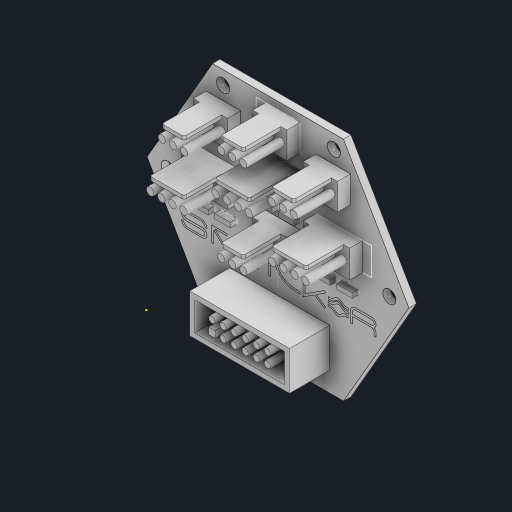
# Autodesk Inventor part: ArmControlBoardPcb
Saved by Autodesk Inventor 2023 (Build 270158000, 158)
## iProperties
Created: 2023-12-09
Part Number: ArmControlBoardPcb
Material: Generic
Document SubType Name: Modeling
Designer: valer
Density: 1 g/cm^3
Appearance: Default
Author: valer
Autodesk Inventor part; units mm, degrees
(part 1 of 3)
ref_plane "YZ Plane" through (0, 0, 0) normal (1, 0, 0) x (0, 1, 0)
ref_plane "XZ Plane" through (0, 0, 0) normal (0, 1, 0) x (-1, 0, 0)
ref_plane "XY Plane" through (0, 0, 0) normal (0, 0, 1) x (1, 0, 0)
sketch "Sketch1" plane through (0, 0, 0) normal (0, 0, 1) x (1, 0, 0)
  circle A0 centre (55.6982, 30.5264) radius 1.5
  line L0 (31.7743, 35.9084) -> (31.7952, 36.0136)
  line L1 (31.7952, 36.0136) -> (31.8548, 36.1028)
  line L2 (31.8548, 36.1028) -> (31.944, 36.1624)
  line L3 (31.944, 36.1624) -> (32.0493, 36.1834)
  line L4 (32.0493, 36.1834) -> (32.7493, 36.1834)
  line L5 (32.7493, 36.1834) -> (32.8545, 36.1624)
  line L6 (32.8545, 36.1624) -> (32.9437, 36.1028)
  line L7 (32.9437, 36.1028) -> (33.0033, 36.0136)
  line L8 (33.0033, 36.0136) -> (33.0243, 35.9084)
  line L9 (33.0243, 35.9084) -> (33.0243, 35.3584)
  line L10 (33.0243, 35.3584) -> (33.0033, 35.2531)
  line L11 (33.0033, 35.2531) -> (32.9437, 35.1639)
  line L12 (32.9437, 35.1639) -> (32.8545, 35.1043)
  line L13 (32.8545, 35.1043) -> (32.7493, 35.0834)
  line L14 (32.7493, 35.0834) -> (32.0493, 35.0834)
  line L15 (32.0493, 35.0834) -> (31.944, 35.1043)
  line L16 (31.944, 35.1043) -> (31.8548, 35.1639)
  line L17 (31.8548, 35.1639) -> (31.7952, 35.2531)
  line L18 (31.7952, 35.2531) -> (31.7743, 35.3584)
  line L19 (31.7743, 35.3584) -> (31.7743, 35.9084)
  line L20 (34.1243, 35.9084) -> (34.1452, 36.0136)
  line L21 (34.1452, 36.0136) -> (34.2048, 36.1028)
  line L22 (34.2048, 36.1028) -> (34.294, 36.1624)
  line L23 (34.294, 36.1624) -> (34.3993, 36.1834)
  line L24 (34.3993, 36.1834) -> (35.0993, 36.1834)
  line L25 (35.0993, 36.1834) -> (35.2045, 36.1624)
  line L26 (35.2045, 36.1624) -> (35.2937, 36.1028)
  line L27 (35.2937, 36.1028) -> (35.3533, 36.0136)
  line L28 (35.3533, 36.0136) -> (35.3743, 35.9084)
  line L29 (35.3743, 35.9084) -> (35.3743, 35.3584)
  line L30 (35.3743, 35.3584) -> (35.3533, 35.2531)
  line L31 (35.3533, 35.2531) -> (35.2937, 35.1639)
  line L32 (35.2937, 35.1639) -> (35.2045, 35.1043)
  line L33 (35.2045, 35.1043) -> (35.0993, 35.0834)
  line L34 (35.0993, 35.0834) -> (34.3993, 35.0834)
  line L35 (34.3993, 35.0834) -> (34.294, 35.1043)
  line L36 (34.294, 35.1043) -> (34.2048, 35.1639)
  line L37 (34.2048, 35.1639) -> (34.1452, 35.2531)
  line L38 (34.1452, 35.2531) -> (34.1243, 35.3584)
  line L39 (34.1243, 35.3584) -> (34.1243, 35.9084)
  line L40 (40.0232, 28.2614) -> (40.0441, 28.3666)
  line L41 (40.0441, 28.3666) -> (40.1037, 28.4558)
  line L42 (40.1037, 28.4558) -> (40.1929, 28.5154)
  line L43 (40.1929, 28.5154) -> (40.2982, 28.5364)
  line L44 (40.2982, 28.5364) -> (40.9982, 28.5364)
  line L45 (40.9982, 28.5364) -> (41.1034, 28.5154)
  line L46 (41.1034, 28.5154) -> (41.1926, 28.4558)
  line L47 (41.1926, 28.4558) -> (41.2522, 28.3666)
  line L48 (41.2522, 28.3666) -> (41.2732, 28.2614)
  line L49 (41.2732, 28.2614) -> (41.2732, 27.7114)
  line L50 (41.2732, 27.7114) -> (41.2522, 27.6061)
  line L51 (41.2522, 27.6061) -> (41.1926, 27.5169)
  line L52 (41.1926, 27.5169) -> (41.1034, 27.4573)
  line L53 (41.1034, 27.4573) -> (40.9982, 27.4364)
  line L54 (40.9982, 27.4364) -> (40.2982, 27.4364)
  line L55 (40.2982, 27.4364) -> (40.1929, 27.4573)
  line L56 (40.1929, 27.4573) -> (40.1037, 27.5169)
  line L57 (40.1037, 27.5169) -> (40.0441, 27.6061)
  line L58 (40.0441, 27.6061) -> (40.0232, 27.7114)
  line L59 (40.0232, 27.7114) -> (40.0232, 28.2614)
  line L60 (42.3732, 28.2614) -> (42.3941, 28.3666)
  line L61 (42.3941, 28.3666) -> (42.4537, 28.4558)
  line L62 (42.4537, 28.4558) -> (42.5429, 28.5154)
  line L63 (42.5429, 28.5154) -> (42.6482, 28.5364)
  line L64 (42.6482, 28.5364) -> (43.3482, 28.5364)
  line L65 (43.3482, 28.5364) -> (43.4534, 28.5154)
  line L66 (43.4534, 28.5154) -> (43.5426, 28.4558)
  line L67 (43.5426, 28.4558) -> (43.6022, 28.3666)
  line L68 (43.6022, 28.3666) -> (43.6232, 28.2614)
  line L69 (43.6232, 28.2614) -> (43.6232, 27.7114)
  line L70 (43.6232, 27.7114) -> (43.6022, 27.6061)
  line L71 (43.6022, 27.6061) -> (43.5426, 27.5169)
  line L72 (43.5426, 27.5169) -> (43.4534, 27.4573)
  line L73 (43.4534, 27.4573) -> (43.3482, 27.4364)
  line L74 (43.3482, 27.4364) -> (42.6482, 27.4364)
  line L75 (42.6482, 27.4364) -> (42.5429, 27.4573)
  line L76 (42.5429, 27.4573) -> (42.4537, 27.5169)
  line L77 (42.4537, 27.5169) -> (42.3941, 27.6061)
  line L78 (42.3941, 27.6061) -> (42.3732, 27.7114)
  line L79 (42.3732, 27.7114) -> (42.3732, 28.2614)
  circle A1 centre (40.4582, 35.6064) radius 0.8763
  circle A2 centre (42.9982, 35.6064) radius 0.8763
  circle A3 centre (45.5382, 35.6064) radius 0.8763
  circle A4 centre (48.0782, 35.6064) radius 0.8763
  line L80 (45.1032, 28.2614) -> (45.1241, 28.3666)
  line L81 (45.1241, 28.3666) -> (45.1837, 28.4558)
  line L82 (45.1837, 28.4558) -> (45.2729, 28.5154)
  line L83 (45.2729, 28.5154) -> (45.3782, 28.5364)
  line L84 (45.3782, 28.5364) -> (46.0782, 28.5364)
  line L85 (46.0782, 28.5364) -> (46.1834, 28.5154)
  line L86 (46.1834, 28.5154) -> (46.2726, 28.4558)
  line L87 (46.2726, 28.4558) -> (46.3322, 28.3666)
  line L88 (46.3322, 28.3666) -> (46.3532, 28.2614)
  line L89 (46.3532, 28.2614) -> (46.3532, 27.7114)
  line L90 (46.3532, 27.7114) -> (46.3322, 27.6061)
  line L91 (46.3322, 27.6061) -> (46.2726, 27.5169)
  line L92 (46.2726, 27.5169) -> (46.1834, 27.4573)
  line L93 (46.1834, 27.4573) -> (46.0782, 27.4364)
  line L94 (46.0782, 27.4364) -> (45.3782, 27.4364)
  line L95 (45.3782, 27.4364) -> (45.2729, 27.4573)
  line L96 (45.2729, 27.4573) -> (45.1837, 27.5169)
  line L97 (45.1837, 27.5169) -> (45.1241, 27.6061)
  line L98 (45.1241, 27.6061) -> (45.1032, 27.7114)
  line L99 (45.1032, 27.7114) -> (45.1032, 28.2614)
  line L100 (47.4532, 28.2614) -> (47.4741, 28.3666)
  line L101 (47.4741, 28.3666) -> (47.5337, 28.4558)
  line L102 (47.5337, 28.4558) -> (47.6229, 28.5154)
  line L103 (47.6229, 28.5154) -> (47.7282, 28.5364)
  line L104 (47.7282, 28.5364) -> (48.4282, 28.5364)
  line L105 (48.4282, 28.5364) -> (48.5334, 28.5154)
  line L106 (48.5334, 28.5154) -> (48.6226, 28.4558)
  line L107 (48.6226, 28.4558) -> (48.6822, 28.3666)
  line L108 (48.6822, 28.3666) -> (48.7032, 28.2614)
  line L109 (48.7032, 28.2614) -> (48.7032, 27.7114)
  line L110 (48.7032, 27.7114) -> (48.6822, 27.6061)
  line L111 (48.6822, 27.6061) -> (48.6226, 27.5169)
  line L112 (48.6226, 27.5169) -> (48.5334, 27.4573)
  line L113 (48.5334, 27.4573) -> (48.4282, 27.4364)
  line L114 (48.4282, 27.4364) -> (47.7282, 27.4364)
  line L115 (47.7282, 27.4364) -> (47.6229, 27.4573)
  line L116 (47.6229, 27.4573) -> (47.5337, 27.5169)
  line L117 (47.5337, 27.5169) -> (47.4741, 27.6061)
  line L118 (47.4741, 27.6061) -> (47.4532, 27.7114)
  line L119 (47.4532, 27.7114) -> (47.4532, 28.2614)
  line L120 (28.5429, 6.4763) -> (28.5638, 6.5815)
  line L121 (28.5638, 6.5815) -> (28.6234, 6.6707)
  line L122 (28.6234, 6.6707) -> (28.7126, 6.7303)
  line L123 (28.7126, 6.7303) -> (28.8179, 6.7513)
  line L124 (28.8179, 6.7513) -> (29.5179, 6.7513)
  line L125 (29.5179, 6.7513) -> (29.6231, 6.7303)
  line L126 (29.6231, 6.7303) -> (29.7123, 6.6707)
  line L127 (29.7123, 6.6707) -> (29.7719, 6.5815)
  line L128 (29.7719, 6.5815) -> (29.7929, 6.4763)
  line L129 (29.7929, 6.4763) -> (29.7929, 5.9263)
  line L130 (29.7929, 5.9263) -> (29.7719, 5.821)
  line L131 (29.7719, 5.821) -> (29.7123, 5.7318)
  line L132 (29.7123, 5.7318) -> (29.6231, 5.6722)
  line L133 (29.6231, 5.6722) -> (29.5179, 5.6513)
  line L134 (29.5179, 5.6513) -> (28.8179, 5.6513)
  line L135 (28.8179, 5.6513) -> (28.7126, 5.6722)
  line L136 (28.7126, 5.6722) -> (28.6234, 5.7318)
  line L137 (28.6234, 5.7318) -> (28.5638, 5.821)
  line L138 (28.5638, 5.821) -> (28.5429, 5.9263)
  line L139 (28.5429, 5.9263) -> (28.5429, 6.4763)
  line L140 (30.8929, 6.4763) -> (30.9138, 6.5815)
  line L141 (30.9138, 6.5815) -> (30.9734, 6.6707)
  line L142 (30.9734, 6.6707) -> (31.0626, 6.7303)
  line L143 (31.0626, 6.7303) -> (31.1679, 6.7513)
  line L144 (31.1679, 6.7513) -> (31.8679, 6.7513)
  line L145 (31.8679, 6.7513) -> (31.9731, 6.7303)
  line L146 (31.9731, 6.7303) -> (32.0623, 6.6707)
  line L147 (32.0623, 6.6707) -> (32.1219, 6.5815)
  line L148 (32.1219, 6.5815) -> (32.1429, 6.4763)
  line L149 (32.1429, 6.4763) -> (32.1429, 5.9263)
  line L150 (32.1429, 5.9263) -> (32.1219, 5.821)
  line L151 (32.1219, 5.821) -> (32.0623, 5.7318)
  line L152 (32.0623, 5.7318) -> (31.9731, 5.6722)
  line L153 (31.9731, 5.6722) -> (31.8679, 5.6513)
  line L154 (31.8679, 5.6513) -> (31.1679, 5.6513)
  line L155 (31.1679, 5.6513) -> (31.0626, 5.6722)
  line L156 (31.0626, 5.6722) -> (30.9734, 5.7318)
  line L157 (30.9734, 5.7318) -> (30.9138, 5.821)
  line L158 (30.9138, 5.821) -> (30.8929, 5.9263)
  line L159 (30.8929, 5.9263) -> (30.8929, 6.4763)
  circle A5 centre (27.4699, 42.6062) radius 0.8763
  circle A6 centre (30.0099, 42.6062) radius 0.8763
  circle A7 centre (32.5499, 42.6062) radius 0.8763
  circle A8 centre (35.0899, 42.6062) radius 0.8763
  circle A9 centre (40.3371, 47.4317) radius 0.8509
  circle A10 centre (42.8771, 47.4317) radius 0.8509
  circle A11 centre (45.4171, 47.4317) radius 0.8509
  line L160 (23.5019, 11.5158) -> (23.5019, 13.0058)
  line L161 (23.5019, 13.0058) -> (24.9919, 13.0058)
  line L162 (24.9919, 13.0058) -> (24.9919, 11.5158)
  line L163 (24.9919, 11.5158) -> (23.5019, 11.5158)
  circle A12 centre (24.2469, 14.8008) radius 0.745
  circle A13 centre (26.7869, 12.2608) radius 0.745
  circle A14 centre (26.7869, 14.8008) radius 0.745
  circle A15 centre (29.3269, 12.2608) radius 0.745
  circle A16 centre (29.3269, 14.8008) radius 0.745
  circle A17 centre (31.8669, 12.2608) radius 0.745
  circle A18 centre (31.8669, 14.8008) radius 0.745
  circle A19 centre (34.4069, 12.2608) radius 0.745
  circle A20 centre (34.4069, 14.8008) radius 0.745
  circle A21 centre (36.9469, 12.2608) radius 0.745
  circle A22 centre (36.9469, 14.8008) radius 0.745
  line L164 (12.0832, 28.2614) -> (12.1041, 28.3666) construction
  line L165 (12.1041, 28.3666) -> (12.1637, 28.4558) construction
  line L166 (12.1637, 28.4558) -> (12.2529, 28.5154) construction
  line L167 (12.2529, 28.5154) -> (12.3582, 28.5364) construction
  line L168 (12.3582, 28.5364) -> (13.0582, 28.5364) construction
  line L169 (13.0582, 28.5364) -> (13.1634, 28.5154) construction
  line L170 (13.1634, 28.5154) -> (13.2526, 28.4558) construction
  line L171 (13.2526, 28.4558) -> (13.3122, 28.3666) construction
  line L172 (13.3122, 28.3666) -> (13.3332, 28.2614) construction
  line L173 (13.3332, 28.2614) -> (13.3332, 27.7114) construction
  line L174 (13.3332, 27.7114) -> (13.3122, 27.6061) construction
  line L175 (13.3122, 27.6061) -> (13.2526, 27.5169) construction
  line L176 (13.2526, 27.5169) -> (13.1634, 27.4573) construction
  line L177 (13.1634, 27.4573) -> (13.0582, 27.4364) construction
  line L178 (13.0582, 27.4364) -> (12.3582, 27.4364) construction
  line L179 (12.3582, 27.4364) -> (12.2529, 27.4573) construction
  line L180 (12.2529, 27.4573) -> (12.1637, 27.5169) construction
  line L181 (12.1637, 27.5169) -> (12.1041, 27.6061) construction
  line L182 (12.1041, 27.6061) -> (12.0832, 27.7114) construction
  line L183 (12.0832, 27.7114) -> (12.0832, 28.2614) construction
  line L184 (14.4332, 28.2614) -> (14.4541, 28.3666) construction
  line L185 (14.4541, 28.3666) -> (14.5137, 28.4558) construction
  line L186 (14.5137, 28.4558) -> (14.6029, 28.5154) construction
  line L187 (14.6029, 28.5154) -> (14.7082, 28.5364) construction
  line L188 (14.7082, 28.5364) -> (15.4082, 28.5364) construction
  line L189 (15.4082, 28.5364) -> (15.5134, 28.5154) construction
  line L190 (15.5134, 28.5154) -> (15.6026, 28.4558) construction
  line L191 (15.6026, 28.4558) -> (15.6622, 28.3666) construction
  line L192 (15.6622, 28.3666) -> (15.6832, 28.2614) construction
  line L193 (15.6832, 28.2614) -> (15.6832, 27.7114) construction
  line L194 (15.6832, 27.7114) -> (15.6622, 27.6061) construction
  line L195 (15.6622, 27.6061) -> (15.6026, 27.5169) construction
  line L196 (15.6026, 27.5169) -> (15.5134, 27.4573) construction
  line L197 (15.5134, 27.4573) -> (15.4082, 27.4364) construction
  line L198 (15.4082, 27.4364) -> (14.7082, 27.4364) construction
  line L199 (14.7082, 27.4364) -> (14.6029, 27.4573) construction
  line L200 (14.6029, 27.4573) -> (14.5137, 27.5169) construction
  line L201 (14.5137, 27.5169) -> (14.4541, 27.6061) construction
  line L202 (14.4541, 27.6061) -> (14.4332, 27.7114) construction
  line L203 (14.4332, 27.7114) -> (14.4332, 28.2614) construction
  circle A23 centre (28.7399, 51.8275) radius 0.8509
  circle A24 centre (31.2799, 51.8275) radius 0.8509
  circle A25 centre (33.8199, 51.8275) radius 0.8509
  line L204 (17.1632, 28.2614) -> (17.1841, 28.3666) construction
  line L205 (17.1841, 28.3666) -> (17.2437, 28.4558) construction
  line L206 (17.2437, 28.4558) -> (17.3329, 28.5154) construction
  line L207 (17.3329, 28.5154) -> (17.4382, 28.5364) construction
  line L208 (17.4382, 28.5364) -> (18.1382, 28.5364)
  line L209 (18.1382, 28.5364) -> (18.2434, 28.5154) construction
  line L210 (18.2434, 28.5154) -> (18.3326, 28.4558) construction
  line L211 (18.3326, 28.4558) -> (18.3922, 28.3666) construction
  line L212 (18.3922, 28.3666) -> (18.4132, 28.2614) construction
  line L213 (18.4132, 28.2614) -> (18.4132, 27.7114) construction
  line L214 (18.4132, 27.7114) -> (18.3922, 27.6061) construction
  line L215 (18.3922, 27.6061) -> (18.3326, 27.5169) construction
  line L216 (18.3326, 27.5169) -> (18.2434, 27.4573) construction
  line L217 (18.2434, 27.4573) -> (18.1382, 27.4364) construction
  line L218 (18.1382, 27.4364) -> (17.4382, 27.4364) construction
  line L219 (17.4382, 27.4364) -> (17.3329, 27.4573) construction
  line L220 (17.3329, 27.4573) -> (17.2437, 27.5169) construction
  line L221 (17.2437, 27.5169) -> (17.1841, 27.6061) construction
  line L222 (17.1841, 27.6061) -> (17.1632, 27.7114) construction
  line L223 (17.1632, 27.7114) -> (17.1632, 28.2614) construction
  line L224 (19.5132, 28.2614) -> (19.5341, 28.3666) construction
  line L225 (19.5341, 28.3666) -> (19.5937, 28.4558) construction
  line L226 (19.5937, 28.4558) -> (19.6829, 28.5154) construction
  line L227 (19.6829, 28.5154) -> (19.7882, 28.5364) construction
  line L228 (19.7882, 28.5364) -> (20.4882, 28.5364) construction
  line L229 (20.4882, 28.5364) -> (20.5934, 28.5154) construction
  line L230 (20.5934, 28.5154) -> (20.6826, 28.4558) construction
  line L231 (20.6826, 28.4558) -> (20.7422, 28.3666) construction
  line L232 (20.7422, 28.3666) -> (20.7632, 28.2614) construction
  line L233 (20.7632, 28.2614) -> (20.7632, 27.7114) construction
  line L234 (20.7632, 27.7114) -> (20.7422, 27.6061) construction
  line L235 (20.7422, 27.6061) -> (20.6826, 27.5169) construction
  line L236 (20.6826, 27.5169) -> (20.5934, 27.4573) construction
  line L237 (20.5934, 27.4573) -> (20.4882, 27.4364) construction
  line L238 (20.4882, 27.4364) -> (19.7882, 27.4364) construction
  line L239 (19.7882, 27.4364) -> (19.6829, 27.4573) construction
  line L240 (19.6829, 27.4573) -> (19.5937, 27.5169) construction
  line L241 (19.5937, 27.5169) -> (19.5341, 27.6061) construction
  line L242 (19.5341, 27.6061) -> (19.5132, 27.7114) construction
  line L243 (19.5132, 27.7114) -> (19.5132, 28.2614) construction
  circle A26 centre (28.7399, 30.5264) radius 0.8509
  circle A27 centre (31.2799, 30.5264) radius 0.8509
  circle A28 centre (33.8199, 30.5264) radius 0.8509
  line L244 (29.4649, 26.3259) -> (29.4858, 26.4311)
  line L245 (29.4858, 26.4311) -> (29.5454, 26.5203)
  line L246 (29.5454, 26.5203) -> (29.6346, 26.5799)
  line L247 (29.6346, 26.5799) -> (29.7399, 26.6009)
  line L248 (29.7399, 26.6009) -> (30.4399, 26.6009)
  line L249 (30.4399, 26.6009) -> (30.5451, 26.5799)
  line L250 (30.5451, 26.5799) -> (30.6343, 26.5203)
  line L251 (30.6343, 26.5203) -> (30.6939, 26.4311)
  line L252 (30.6939, 26.4311) -> (30.7149, 26.3259)
  line L253 (30.7149, 26.3259) -> (30.7149, 25.7759)
  line L254 (30.7149, 25.7759) -> (30.6939, 25.6706)
  line L255 (30.6939, 25.6706) -> (30.6343, 25.5814)
  line L256 (30.6343, 25.5814) -> (30.5451, 25.5218)
  line L257 (30.5451, 25.5218) -> (30.4399, 25.5009)
  line L258 (30.4399, 25.5009) -> (29.7399, 25.5009)
  line L259 (29.7399, 25.5009) -> (29.6346, 25.5218)
  line L260 (29.6346, 25.5218) -> (29.5454, 25.5814)
  line L261 (29.5454, 25.5814) -> (29.4858, 25.6706)
  line L262 (29.4858, 25.6706) -> (29.4649, 25.7759)
  line L263 (29.4649, 25.7759) -> (29.4649, 26.3259)
  line L264 (31.8149, 26.3259) -> (31.8358, 26.4311)
  line L265 (31.8358, 26.4311) -> (31.8954, 26.5203)
  line L266 (31.8954, 26.5203) -> (31.9846, 26.5799)
  line L267 (31.9846, 26.5799) -> (32.0899, 26.6009)
  line L268 (32.0899, 26.6009) -> (32.7899, 26.6009)
  line L269 (32.7899, 26.6009) -> (32.8951, 26.5799)
  line L270 (32.8951, 26.5799) -> (32.9843, 26.5203)
  line L271 (32.9843, 26.5203) -> (33.0439, 26.4311)
  line L272 (33.0439, 26.4311) -> (33.0649, 26.3259)
  line L273 (33.0649, 25.7759) -> (33.0439, 25.6706)
  line L274 (33.0439, 25.6706) -> (32.9843, 25.5814)
  line L275 (32.9843, 25.5814) -> (32.8951, 25.5218)
  line L276 (32.8951, 25.5218) -> (32.7899, 25.5009)
  line L277 (32.7899, 25.5009) -> (32.0899, 25.5009)
  line L278 (32.0899, 25.5009) -> (31.9846, 25.5218)
  line L279 (31.9846, 25.5218) -> (31.8954, 25.5814)
  line L280 (31.8954, 25.5814) -> (31.8358, 25.6706)
  line L281 (31.8358, 25.6706) -> (31.8149, 25.7759)
  line L282 (31.8149, 25.7759) -> (31.8149, 26.3259)
  circle A29 centre (12.5182, 35.6064) radius 0.8763
  circle A30 centre (15.0582, 35.6064) radius 0.8763
  circle A31 centre (17.5982, 35.6064) radius 0.8763
  circle A32 centre (20.1382, 35.6064) radius 0.8763
  line L283 (26.6943, 35.9084) -> (26.7152, 36.0136)
  line L284 (26.7152, 36.0136) -> (26.7748, 36.1028)
  line L285 (26.7748, 36.1028) -> (26.864, 36.1624)
  line L286 (26.864, 36.1624) -> (26.9693, 36.1834)
  line L287 (26.9693, 36.1834) -> (27.6693, 36.1834)
  line L288 (27.6693, 36.1834) -> (27.7745, 36.1624)
  line L289 (27.7745, 36.1624) -> (27.8637, 36.1028)
  line L290 (27.8637, 36.1028) -> (27.9233, 36.0136)
  line L291 (27.9233, 36.0136) -> (27.9443, 35.9084)
  line L292 (27.9443, 35.9084) -> (27.9443, 35.3584)
  line L293 (27.9443, 35.3584) -> (27.9233, 35.2531)
  line L294 (27.9233, 35.2531) -> (27.8637, 35.1639)
  line L295 (27.8637, 35.1639) -> (27.7745, 35.1043)
  line L296 (27.7745, 35.1043) -> (27.6693, 35.0834)
  line L297 (27.6693, 35.0834) -> (26.9693, 35.0834)
  line L298 (26.9693, 35.0834) -> (26.864, 35.1043)
  line L299 (26.864, 35.1043) -> (26.7748, 35.1639)
  line L300 (26.7748, 35.1639) -> (26.7152, 35.2531)
  line L301 (26.7152, 35.2531) -> (26.6943, 35.3584)
  line L302 (26.6943, 35.3584) -> (26.6943, 35.9084)
  line L303 (29.0443, 35.9084) -> (29.0652, 36.0136)
  line L304 (29.0652, 36.0136) -> (29.1248, 36.1028)
  line L305 (29.1248, 36.1028) -> (29.214, 36.1624)
  line L306 (29.214, 36.1624) -> (29.3193, 36.1834)
  line L307 (29.3193, 36.1834) -> (30.0193, 36.1834)
  line L308 (30.0193, 36.1834) -> (30.1245, 36.1624)
  line L309 (30.1245, 36.1624) -> (30.2137, 36.1028)
  line L310 (30.2137, 36.1028) -> (30.2733, 36.0136)
  line L311 (30.2733, 36.0136) -> (30.2943, 35.9084)
  line L312 (30.2943, 35.9084) -> (30.2943, 35.3584)
  line L313 (30.2943, 35.3584) -> (30.2733, 35.2531)
  line L314 (30.2733, 35.2531) -> (30.2137, 35.1639)
  line L315 (30.2137, 35.1639) -> (30.1245, 35.1043)
  line L316 (30.1245, 35.1043) -> (30.0193, 35.0834)
  line L317 (30.0193, 35.0834) -> (29.3193, 35.0834)
  line L318 (29.3193, 35.0834) -> (29.214, 35.1043)
  line L319 (29.214, 35.1043) -> (29.1248, 35.1639)
  line L320 (29.1248, 35.1639) -> (29.0652, 35.2531)
  line L321 (29.0652, 35.2531) -> (29.0443, 35.3584)
  line L322 (29.0443, 35.3584) -> (29.0443, 35.9084)
  circle A33 centre (15.1689, 47.3537) radius 0.8509
  circle A34 centre (17.7089, 47.3537) radius 0.8509
  circle A35 centre (20.2489, 47.3537) radius 0.8509
  line L323 (20.1652, 35.6334) -> (20.1382, 35.6064)
  line L324 (26.4028, 18.3787) -> (26.4027, 18.3787)
  line L325 (44.019, 24.3143) -> (44.055, 24.3125)
  line L326 (44.055, 24.3125) -> (44.0904, 24.3095)
  line L327 (44.0904, 24.3095) -> (44.125, 24.3055)
  line L328 (44.125, 24.3055) -> (44.159, 24.3003)
  line L329 (44.159, 24.3003) -> (44.1923, 24.2942)
  line L330 (44.1923, 24.2942) -> (44.257, 24.2789)
  line L331 (44.257, 24.2789) -> (44.3195, 24.2602)
  line L332 (44.3195, 24.2602) -> (44.3798, 24.2382)
  line L333 (44.3798, 24.2382) -> (44.4381, 24.2133)
  line L334 (44.4381, 24.2133) -> (44.4948, 24.1859)
  line L335 (44.4948, 24.1859) -> (44.5498, 24.1564)
  line L336 (44.5498, 24.1564) -> (44.6035, 24.125)
  line L337 (44.6035, 24.125) -> (44.6561, 24.0922)
  line L338 (44.6561, 24.0922) -> (44.7077, 24.0582)
  line L339 (44.7077, 24.0582) -> (44.8087, 23.9883)
  line L340 (44.8087, 23.9883) -> (44.9082, 23.918)
  line L341 (44.9082, 23.918) -> (45.1198, 23.7816)
  line L342 (45.1198, 23.7816) -> (45.2244, 23.718)
  line L343 (45.2244, 23.718) -> (45.2775, 23.6882)
  line L344 (45.2775, 23.6882) -> (45.3315, 23.6601)
  line L345 (45.3315, 23.6601) -> (45.3867, 23.6337)
  line L346 (45.3867, 23.6337) -> (45.4435, 23.6095)
  line L347 (45.4435, 23.6095) -> (45.5022, 23.5876)
  line L348 (45.5022, 23.5876) -> (45.563, 23.5683)
  line L349 (45.563, 23.5683) -> (45.6263, 23.5517)
  line L350 (45.6263, 23.5517) -> (45.6924, 23.5382)
  line L351 (45.6924, 23.5382) -> (45.7616, 23.5279)
  line L352 (45.7616, 23.5279) -> (45.8342, 23.5212)
  line L353 (45.8342, 23.5212) -> (46.3369, 23.5212)
  line L354 (46.3369, 23.5212) -> (46.3369, 23.0714)
  line L355 (46.3369, 23.0714) -> (45.8342, 23.0714)
  line L356 (45.8342, 23.0714) -> (45.7851, 23.0722)
  line L357 (45.7851, 23.0722) -> (45.7371, 23.0747)
  line L358 (45.7371, 23.0747) -> (45.6902, 23.0787)
  line L359 (45.6902, 23.0787) -> (45.6442, 23.0843)
  line L360 (45.6442, 23.0843) -> (45.5992, 23.0913)
  line L361 (45.5992, 23.0913) -> (45.5552, 23.0996)
  line L362 (45.5552, 23.0996) -> (45.5121, 23.1093)
  line L363 (45.5121, 23.1093) -> (45.47, 23.1202)
  line L364 (45.47, 23.1202) -> (45.4287, 23.1322)
  line L365 (45.4287, 23.1322) -> (45.3883, 23.1453)
  line L366 (45.3883, 23.1453) -> (45.3101, 23.1746)
  line L367 (45.3101, 23.1746) -> (45.2349, 23.2075)
  line L368 (45.2349, 23.2075) -> (45.1628, 23.2433)
  line L369 (45.1628, 23.2433) -> (45.0935, 23.2817)
  line L370 (45.0935, 23.2817) -> (45.0268, 23.322)
  line L371 (45.0268, 23.322) -> (44.9624, 23.3637)
  line L372 (44.9624, 23.3637) -> (44.9003, 23.4062)
  line L373 (44.9003, 23.4062) -> (44.7819, 23.4917)
  line L374 (44.7819, 23.4917) -> (44.67, 23.5741)
  line L375 (44.67, 23.5741) -> (44.583, 23.6409)
  line L376 (44.583, 23.6409) -> (44.4997, 23.7018)
  line L377 (44.4997, 23.7018) -> (44.4591, 23.7298)
  line L378 (44.4591, 23.7298) -> (44.4189, 23.7559)
  line L379 (44.4189, 23.7559) -> (44.379, 23.7801)
  line L380 (44.379, 23.7801) -> (44.3393, 23.8023)
  line L381 (44.3393, 23.8023) -> (44.2996, 23.8223)
  line L382 (44.2996, 23.8223) -> (44.2597, 23.84)
  line L383 (44.2597, 23.84) -> (44.2195, 23.8552)
  line L384 (44.2195, 23.8552) -> (44.1789, 23.868)
  line L385 (44.1789, 23.868) -> (44.1376, 23.8781)
  line L386 (44.1376, 23.8781) -> (44.0956, 23.8855)
  line L387 (44.0956, 23.8855) -> (44.0526, 23.89)
  line L388 (44.0526, 23.89) -> (44.0086, 23.8916)
  line L389 (44.0086, 23.8916) -> (43.9645, 23.89)
  line L390 (43.9645, 23.89) -> (43.9216, 23.8855)
  line L391 (43.9216, 23.8855) -> (43.8795, 23.8781)
  line L392 (43.8795, 23.8781) -> (43.8383, 23.868)
  line L393 (43.8383, 23.868) -> (43.7976, 23.8552)
  line L394 (43.7976, 23.8552) -> (43.7574, 23.84)
  line L395 (43.7574, 23.84) -> (43.7176, 23.8223)
  line L396 (43.7176, 23.8223) -> (43.6779, 23.8023)
  line L397 (43.6779, 23.8023) -> (43.6381, 23.7801)
  line L398 (43.6381, 23.7801) -> (43.5983, 23.7559)
  line L399 (43.5983, 23.7559) -> (43.5581, 23.7298)
  line L400 (43.5581, 23.7298) -> (43.5174, 23.7018)
  line L401 (43.5174, 23.7018) -> (43.4341, 23.6409)
  line L402 (43.4341, 23.6409) -> (43.3471, 23.5741)
  line L403 (43.3471, 23.5741) -> (43.2352, 23.4841)
  line L404 (43.2352, 23.4841) -> (43.1169, 23.3951)
  line L405 (43.1169, 23.3951) -> (43.0547, 23.352)
  line L406 (43.0547, 23.352) -> (42.9904, 23.3104)
  line L407 (42.9904, 23.3104) -> (42.9237, 23.2707)
  line L408 (42.9237, 23.2707) -> (42.8543, 23.2334)
  line L409 (42.8543, 23.2334) -> (42.7822, 23.1989)
  line L410 (42.7822, 23.1989) -> (42.7071, 23.1676)
  line L411 (42.7071, 23.1676) -> (42.6288, 23.14)
  line L412 (42.6288, 23.14) -> (42.5472, 23.1164)
  line L413 (42.5472, 23.1164) -> (42.462, 23.0974)
  line L414 (42.462, 23.0974) -> (42.373, 23.0832)
  line L415 (42.373, 23.0832) -> (42.28, 23.0744)
  line L416 (42.28, 23.0744) -> (42.183, 23.0714)
  line L417 (42.183, 23.0714) -> (41.6803, 23.0714)
  line L418 (41.6803, 23.0714) -> (41.6803, 23.5212)
  line L419 (41.6803, 23.5212) -> (42.183, 23.5212)
  line L420 (42.183, 23.5212) -> (42.215, 23.5218)
  line L421 (42.215, 23.5218) -> (42.2465, 23.5236)
  line L422 (42.2465, 23.5236) -> (42.2777, 23.5265)
  line L423 (42.2777, 23.5265) -> (42.3084, 23.5306)
  line L424 (42.3084, 23.5306) -> (42.3387, 23.5358)
  line L425 (42.3387, 23.5358) -> (42.3686, 23.5419)
  line L426 (42.3686, 23.5419) -> (42.4273, 23.5571)
  line L427 (42.4273, 23.5571) -> (42.4846, 23.5759)
  line L428 (42.4846, 23.5759) -> (42.5406, 23.5979)
  line L429 (42.5406, 23.5979) -> (42.5955, 23.6228)
  line L430 (42.5955, 23.6228) -> (42.6493, 23.6501)
  line L431 (42.6493, 23.6501) -> (42.7022, 23.6797)
  line L432 (42.7022, 23.6797) -> (42.7542, 23.7111)
  line L433 (42.7542, 23.7111) -> (42.8056, 23.7439)
  line L434 (42.8056, 23.7439) -> (42.8564, 23.7779)
  line L435 (42.8564, 23.7779) -> (43.0561, 23.918)
  line L436 (43.0561, 23.918) -> (43.1556, 23.9959)
  line L437 (43.1556, 23.9959) -> (43.2058, 24.0333)
  line L438 (43.2058, 24.0333) -> (43.2566, 24.0693)
  line L439 (43.2566, 24.0693) -> (43.3082, 24.1039)
  line L440 (43.3082, 24.1039) -> (43.3607, 24.1366)
  line L441 (43.3607, 24.1366) -> (43.4144, 24.1674)
  line L442 (43.4144, 24.1674) -> (43.4695, 24.1958)
  line L443 (43.4695, 24.1958) -> (43.5261, 24.2219)
  line L444 (43.5261, 24.2219) -> (43.5845, 24.2451)
  line L445 (43.5845, 24.2451) -> (43.6448, 24.2655)
  line L446 (43.6448, 24.2655) -> (43.7072, 24.2827)
  line L447 (43.7072, 24.2827) -> (43.772, 24.2964)
  line L448 (43.772, 24.2964) -> (43.8392, 24.3065)
  line L449 (43.8392, 24.3065) -> (43.9092, 24.3128)
  line L450 (43.9092, 24.3128) -> (43.9821, 24.3149)
  line L451 (43.9821, 24.3149) -> (44.019, 24.3143)
  line L452 (18.5028, 23.971) -> (15.7246, 23.971)
  line L453 (15.7246, 23.971) -> (18.635, 21.087)
  line L454 (18.635, 21.087) -> (18.344, 20.7695)
  line L455 (18.344, 20.7695) -> (15.4336, 23.6535)
  line L456 (15.4336, 23.6535) -> (15.4336, 20.8753)
  line L457 (15.4336, 20.8753) -> (14.9838, 20.8753)
  line L458 (14.9838, 20.8753) -> (14.9838, 24.3943)
  line L459 (14.9838, 24.3943) -> (18.5028, 24.3943)
  line L460 (18.5028, 24.3943) -> (18.5028, 23.971)
  line L461 (51.3988, 24.4192) -> (51.4835, 24.4146)
  line L462 (51.4835, 24.4146) -> (51.5652, 24.407)
  line L463 (51.5652, 24.407) -> (51.6439, 24.3964)
  line L464 (51.6439, 24.3964) -> (51.7196, 24.3828)
  line L465 (51.7196, 24.3828) -> (51.7925, 24.3663)
  line L466 (51.7925, 24.3663) -> (51.8624, 24.347)
  line L467 (51.8624, 24.347) -> (51.9295, 24.3248)
  line L468 (51.9295, 24.3248) -> (51.9939, 24.2999)
  line L469 (51.9939, 24.2999) -> (52.0555, 24.2722)
  line L470 (52.0555, 24.2722) -> (52.1144, 24.2418)
  line L471 (52.1144, 24.2418) -> (52.1706, 24.2087)
  line L472 (52.1706, 24.2087) -> (52.2241, 24.1729)
  line L473 (52.2241, 24.1729) -> (52.2751, 24.1346)
  line L474 (52.2751, 24.1346) -> (52.3235, 24.0937)
  line L475 (52.3235, 24.0937) -> (52.3694, 24.0503)
  line L476 (52.3694, 24.0503) -> (52.3935, 24.0254)
  line L477 (52.3935, 24.0254) -> (52.416, 24.0002)
  line L478 (52.416, 24.0002) -> (52.4371, 23.9748)
  line L479 (52.4371, 23.9748) -> (52.4567, 23.9493)
  line L480 (52.4567, 23.9493) -> (52.4751, 23.9237)
  line L481 (52.4751, 23.9237) -> (52.4921, 23.8982)
  line L482 (52.4921, 23.8982) -> (52.5078, 23.8727)
  line L483 (52.5078, 23.8727) -> (52.5224, 23.8473)
  line L484 (52.5224, 23.8473) -> (52.5358, 23.8222)
  line L485 (52.5358, 23.8222) -> (52.548, 23.7973)
  line L486 (52.548, 23.7973) -> (52.5592, 23.7727)
  line L487 (52.5592, 23.7727) -> (52.5694, 23.7485)
  line L488 (52.5694, 23.7485) -> (52.5869, 23.7015)
  line L489 (52.5869, 23.7015) -> (52.6009, 23.6568)
  line L490 (52.6009, 23.6568) -> (52.6118, 23.6148)
  line L491 (52.6118, 23.6148) -> (52.62, 23.5762)
  line L492 (52.62, 23.5762) -> (52.6259, 23.5414)
  line L493 (52.6259, 23.5414) -> (52.6299, 23.5108)
  line L494 (52.6299, 23.5108) -> (52.6323, 23.4851)
  line L495 (52.6323, 23.4851) -> (52.6335, 23.4647)
  line L496 (52.6335, 23.4647) -> (52.634, 23.4418)
  line L497 (52.634, 23.4418) -> (52.634, 23.336)
  line L498 (52.634, 23.336) -> (52.6299, 23.2785)
  line L499 (52.6299, 23.2785) -> (52.6259, 23.2489)
  line L500 (52.6259, 23.2489) -> (52.62, 23.2146)
  line L501 (52.62, 23.2146) -> (52.6118, 23.1761)
  line L502 (52.6118, 23.1761) -> (52.6009, 23.1342)
  line L503 (52.6009, 23.1342) -> (52.5869, 23.0895)
  line L504 (52.5869, 23.0895) -> (52.5694, 23.0427)
  line L505 (52.5694, 23.0427) -> (52.548, 22.9944)
  line L506 (52.548, 22.9944) -> (52.5224, 22.9453)
  line L507 (52.5224, 22.9453) -> (52.4921, 22.896)
  line L508 (52.4921, 22.896) -> (52.4751, 22.8715)
  line L509 (52.4751, 22.8715) -> (52.4567, 22.8472)
  line L510 (52.4567, 22.8472) -> (52.4371, 22.8233)
  line L511 (52.4371, 22.8233) -> (52.416, 22.7996)
  line L512 (52.416, 22.7996) -> (52.3935, 22.7765)
  line L513 (52.3935, 22.7765) -> (52.3694, 22.7539)
  line L514 (52.3694, 22.7539) -> (52.3293, 22.7142)
  line L515 (52.3293, 22.7142) -> (52.3085, 22.6943)
  line L516 (52.3085, 22.6943) -> (52.2867, 22.6745)
  line L517 (52.2867, 22.6745) -> (52.2637, 22.6546)
  line L518 (52.2637, 22.6546) -> (52.2517, 22.6447)
  line L519 (52.2517, 22.6447) -> (52.2392, 22.6348)
  line L520 (52.2392, 22.6348) -> (52.2262, 22.6249)
  line L521 (52.2262, 22.6249) -> (52.2128, 22.615)
  line L522 (52.2128, 22.615) -> (52.1988, 22.605)
  line L523 (52.1988, 22.605) -> (52.1842, 22.5951)
  line L524 (52.1842, 22.5951) -> (52.1988, 22.5852)
  line L525 (52.1988, 22.5852) -> (52.2128, 22.5753)
  line L526 (52.2128, 22.5753) -> (52.2262, 22.5654)
  line L527 (52.2262, 22.5654) -> (52.2392, 22.5554)
  line L528 (52.2392, 22.5554) -> (52.2517, 22.5455)
  line L529 (52.2517, 22.5455) -> (52.2637, 22.5356)
  line L530 (52.2637, 22.5356) -> (52.2754, 22.5257)
  line L531 (52.2754, 22.5257) -> (52.2867, 22.5157)
  line L532 (52.2867, 22.5157) -> (52.3085, 22.4959)
  line L533 (52.3085, 22.4959) -> (52.3293, 22.4761)
  line L534 (52.3293, 22.4761) -> (52.3495, 22.4562)
  line L535 (52.3495, 22.4562) -> (52.3694, 22.4364)
  line L536 (52.3694, 22.4364) -> (52.3935, 22.4114)
  line L537 (52.3935, 22.4114) -> (52.416, 22.3862)
  line L538 (52.416, 22.3862) -> (52.4371, 22.3608)
  line L539 (52.4371, 22.3608) -> (52.4567, 22.3353)
  line L540 (52.4567, 22.3353) -> (52.4751, 22.3098)
  line L541 (52.4751, 22.3098) -> (52.4921, 22.2842)
  line L542 (52.4921, 22.2842) -> (52.5078, 22.2587)
  line L543 (52.5078, 22.2587) -> (52.5224, 22.2334)
  line L544 (52.5224, 22.2334) -> (52.5358, 22.2082)
  line L545 (52.5358, 22.2082) -> (52.548, 22.1833)
  line L546 (52.548, 22.1833) -> (52.5592, 22.1587)
  line L547 (52.5592, 22.1587) -> (52.5694, 22.1345)
  line L548 (52.5694, 22.1345) -> (52.5869, 22.0875)
  line L549 (52.5869, 22.0875) -> (52.6009, 22.0428)
  line L550 (52.6009, 22.0428) -> (52.6118, 22.0009)
  line L551 (52.6118, 22.0009) -> (52.62, 21.9622)
  line L552 (52.62, 21.9622) -> (52.6259, 21.9274)
  line L553 (52.6259, 21.9274) -> (52.6299, 21.8969)
  line L554 (52.6299, 21.8969) -> (52.6323, 21.8711)
  line L555 (52.6323, 21.8711) -> (52.6335, 21.8507)
  line L556 (52.6335, 21.8507) -> (52.634, 21.8278)
  line L557 (52.634, 21.8278) -> (52.634, 20.8753)
  line L558 (52.634, 20.8753) -> (52.1842, 20.8753)
  line L559 (52.1842, 20.8753) -> (52.1842, 21.8278)
  line L560 (52.1842, 21.8278) -> (52.1825, 21.8658)
  line L561 (52.1825, 21.8658) -> (52.1785, 21.8963)
  line L562 (52.1785, 21.8963) -> (52.1706, 21.9328)
  line L563 (52.1706, 21.9328) -> (52.1576, 21.974)
  line L564 (52.1576, 21.974) -> (52.1382, 22.0185)
  line L565 (52.1382, 22.0185) -> (52.1111, 22.065)
  line L566 (52.1111, 22.065) -> (52.0943, 22.0886)
  line L567 (52.0943, 22.0886) -> (52.0751, 22.1123)
  line L568 (52.0751, 22.1123) -> (52.0533, 22.1357)
  line L569 (52.0533, 22.1357) -> (52.0288, 22.1589)
  line L570 (52.0288, 22.1589) -> (52.0014, 22.1815)
  line L571 (52.0014, 22.1815) -> (51.971, 22.2035)
  line L572 (51.971, 22.2035) -> (51.9374, 22.2247)
  line L573 (51.9374, 22.2247) -> (51.9005, 22.2449)
  line L574 (51.9005, 22.2449) -> (51.86, 22.264)
  line L575 (51.86, 22.264) -> (51.8159, 22.2818)
  line L576 (51.8159, 22.2818) -> (51.7679, 22.298)
  line L577 (51.7679, 22.298) -> (51.7159, 22.3127)
  line L578 (51.7159, 22.3127) -> (51.6597, 22.3255)
  line L579 (51.6597, 22.3255) -> (51.5993, 22.3364)
  line L580 (51.5993, 22.3364) -> (51.5343, 22.3452)
  line L581 (51.5343, 22.3452) -> (51.4648, 22.3516)
  line L582 (51.4648, 22.3516) -> (51.3904, 22.3556)
  line L583 (51.3904, 22.3556) -> (51.3111, 22.357)
  line L584 (51.3111, 22.357) -> (47.263, 22.357)
  line L585 (47.263, 22.357) -> (47.263, 20.8753)
  line L586 (47.263, 20.8753) -> (46.8132, 20.8753)
  line L587 (46.8132, 20.8753) -> (46.8132, 22.8068)
  line L588 (47.263, 22.8068) -> (51.3111, 22.8068)
  line L589 (51.3111, 22.8068) -> (51.3743, 22.8074)
  line L590 (51.3743, 22.8074) -> (51.4352, 22.8094)
  line L591 (51.4352, 22.8094) -> (51.4936, 22.8127)
  line L592 (51.4936, 22.8127) -> (51.5496, 22.8175)
  line L593 (51.5496, 22.8175) -> (51.6033, 22.8239)
  line L594 (51.6033, 22.8239) -> (51.6548, 22.8319)
  line L595 (51.6548, 22.8319) -> (51.704, 22.8416)
  line L596 (51.704, 22.8416) -> (51.751, 22.8531)
  line L597 (51.751, 22.8531) -> (51.7958, 22.8664)
  line L598 (51.7958, 22.8664) -> (51.8384, 22.8817)
  line L599 (51.8384, 22.8817) -> (51.879, 22.899)
  line L600 (51.879, 22.899) -> (51.9176, 22.9184)
  line L601 (51.9176, 22.9184) -> (51.9541, 22.94)
  line L602 (51.9541, 22.94) -> (51.9886, 22.9638)
  line L603 (51.9886, 22.9638) -> (52.0212, 22.9899)
  line L604 (52.0212, 22.9899) -> (52.0519, 23.0185)
  line L605 (52.0519, 23.0185) -> (52.0663, 23.0286)
  line L606 (52.0663, 23.0286) -> (52.0799, 23.0392)
  line L607 (52.0799, 23.0392) -> (52.0925, 23.0501)
  line L608 (52.0925, 23.0501) -> (52.1043, 23.0613)
  line L609 (52.1043, 23.0613) -> (52.1153, 23.0729)
  line L610 (52.1153, 23.0729) -> (52.1255, 23.0846)
  line L611 (52.1255, 23.0846) -> (52.135, 23.0965)
  line L612 (52.135, 23.0965) -> (52.1437, 23.1086)
  line L613 (52.1437, 23.1086) -> (52.1517, 23.1207)
  line L614 (52.1517, 23.1207) -> (52.1591, 23.1328)
  line L615 (52.1591, 23.1328) -> (52.1658, 23.145)
  line L616 (52.1658, 23.145) -> (52.1719, 23.157)
  line L617 (52.1719, 23.157) -> (52.1774, 23.169)
  line L618 (52.1774, 23.169) -> (52.1824, 23.1808)
  line L619 (52.1824, 23.1808) -> (52.1869, 23.1924)
  line L620 (52.1869, 23.1924) -> (52.1908, 23.2037)
  line L621 (52.1908, 23.2037) -> (52.1974, 23.2253)
  line L622 (52.1974, 23.2253) -> (52.2023, 23.2453)
  line L623 (52.2023, 23.2453) -> (52.2058, 23.2633)
  line L624 (52.2058, 23.2633) -> (52.2082, 23.2789)
  line L625 (52.2082, 23.2789) -> (52.2096, 23.2917)
  line L626 (52.2096, 23.2917) -> (52.2104, 23.3013)
  line L627 (52.2104, 23.3013) -> (52.2107, 23.3095)
  line L628 (52.2107, 23.3095) -> (52.2107, 23.4153)
  line L629 (52.2107, 23.4153) -> (52.209, 23.4533)
  line L630 (52.209, 23.4533) -> (52.2049, 23.4838)
  line L631 (52.2049, 23.4838) -> (52.197, 23.5203)
  line L632 (52.197, 23.5203) -> (52.184, 23.5615)
  line L633 (52.184, 23.5615) -> (52.1646, 23.606)
  line L634 (52.1646, 23.606) -> (52.1376, 23.6525)
  line L635 (52.1376, 23.6525) -> (52.1207, 23.6761)
  line L636 (52.1207, 23.6761) -> (52.1015, 23.6998)
  line L637 (52.1015, 23.6998) -> (52.0798, 23.7232)
  line L638 (52.0798, 23.7232) -> (52.0553, 23.7464)
  line L639 (52.0553, 23.7464) -> (52.0279, 23.769)
  line L640 (52.0279, 23.769) -> (51.9975, 23.791)
  line L641 (51.9975, 23.791) -> (51.9639, 23.8122)
  line L642 (51.9639, 23.8122) -> (51.9269, 23.8324)
  line L643 (51.9269, 23.8324) -> (51.8865, 23.8515)
  line L644 (51.8865, 23.8515) -> (51.8423, 23.8693)
  line L645 (51.8423, 23.8693) -> (51.7943, 23.8855)
  line L646 (51.7943, 23.8855) -> (51.7423, 23.9002)
  line L647 (51.7423, 23.9002) -> (51.6862, 23.913)
  line L648 (51.6862, 23.913) -> (51.6257, 23.9239)
  line L649 (51.6257, 23.9239) -> (51.5608, 23.9327)
  line L650 (51.5608, 23.9327) -> (51.4912, 23.9391)
  line L651 (51.4912, 23.9391) -> (51.4169, 23.9431)
  line L652 (51.4169, 23.9431) -> (51.3375, 23.9445)
  line L653 (51.3375, 23.9445) -> (48.1625, 23.9445)
  line L654 (48.1625, 23.9445) -> (48.0993, 23.9439)
  line L655 (48.0993, 23.9439) -> (48.0385, 23.9419)
  line L656 (48.0385, 23.9419) -> (47.9801, 23.9386)
  line L657 (47.9801, 23.9386) -> (47.924, 23.9337)
  line L658 (47.924, 23.9337) -> (47.8703, 23.9274)
  line L659 (47.8703, 23.9274) -> (47.8188, 23.9194)
  line L660 (47.8188, 23.9194) -> (47.7697, 23.9097)
  line L661 (47.7697, 23.9097) -> (47.7227, 23.8982)
  line L662 (47.7227, 23.8982) -> (47.6779, 23.8848)
  line L663 (47.6779, 23.8848) -> (47.6352, 23.8696)
  line L664 (47.6352, 23.8696) -> (47.5946, 23.8523)
  line L665 (47.5946, 23.8523) -> (47.5561, 23.8329)
  line L666 (47.5561, 23.8329) -> (47.5196, 23.8113)
  line L667 (47.5196, 23.8113) -> (47.485, 23.7875)
  line L668 (47.485, 23.7875) -> (47.4524, 23.7614)
  line L669 (47.4524, 23.7614) -> (47.4217, 23.7328)
  line L670 (47.4217, 23.7328) -> (47.4073, 23.7227)
  line L671 (47.4073, 23.7227) -> (47.3938, 23.7121)
  line L672 (47.3938, 23.7121) -> (47.3811, 23.7012)
  line L673 (47.3811, 23.7012) -> (47.3693, 23.6899)
  line L674 (47.3693, 23.6899) -> (47.3583, 23.6784)
  line L675 (47.3583, 23.6784) -> (47.3481, 23.6667)
  line L676 (47.3481, 23.6667) -> (47.3387, 23.6547)
  line L677 (47.3387, 23.6547) -> (47.3299, 23.6427)
  line L678 (47.3299, 23.6427) -> (47.3219, 23.6306)
  line L679 (47.3219, 23.6306) -> (47.3145, 23.6184)
  line L680 (47.3145, 23.6184) -> (47.3078, 23.6063)
  line L681 (47.3078, 23.6063) -> (47.3017, 23.5942)
  line L682 (47.3017, 23.5942) -> (47.2962, 23.5823)
  line L683 (47.2962, 23.5823) -> (47.2912, 23.5705)
  line L684 (47.2912, 23.5705) -> (47.2868, 23.5589)
  line L685 (47.2868, 23.5589) -> (47.2828, 23.5476)
  line L686 (47.2828, 23.5476) -> (47.2763, 23.526)
  line L687 (47.2763, 23.526) -> (47.2713, 23.506)
  line L688 (47.2713, 23.506) -> (47.2678, 23.488)
  line L689 (47.2678, 23.488) -> (47.2654, 23.4724)
  line L690 (47.2654, 23.4724) -> (47.264, 23.4596)
  line L691 (47.264, 23.4596) -> (47.2633, 23.4499)
  line L692 (47.2633, 23.4499) -> (47.263, 23.4418)
  line L693 (47.263, 23.4418) -> (47.263, 22.8068)
  line L694 (46.8132, 22.8068) -> (46.8132, 23.4418)
  line L695 (46.8132, 23.4418) -> (46.8173, 23.4997)
  line L696 (46.8173, 23.4997) -> (46.8271, 23.5646)
  line L697 (46.8271, 23.5646) -> (46.8353, 23.6038)
  line L698 (46.8353, 23.6038) -> (46.8462, 23.6468)
  line L699 (46.8462, 23.6468) -> (46.8603, 23.6929)
  line L700 (46.8603, 23.6929) -> (46.8778, 23.7415)
  line L701 (46.8778, 23.7415) -> (46.8991, 23.7919)
  line L702 (46.8991, 23.7919) -> (46.9248, 23.8436)
  line L703 (46.9248, 23.8436) -> (46.9551, 23.8959)
  line L704 (46.9551, 23.8959) -> (46.9904, 23.9482)
  line L705 (46.9904, 23.9482) -> (47.0101, 23.9742)
  line L706 (47.0101, 23.9742) -> (47.0312, 23.9999)
  line L707 (47.0312, 23.9999) -> (47.0537, 24.0253)
  line L708 (47.0537, 24.0253) -> (47.0778, 24.0503)
  line L709 (47.0778, 24.0503) -> (47.1236, 24.0937)
  line L710 (47.1236, 24.0937) -> (47.1721, 24.1346)
  line L711 (47.1721, 24.1346) -> (47.223, 24.1729)
  line L712 (47.223, 24.1729) -> (47.2766, 24.2087)
  line L713 (47.2766, 24.2087) -> (47.3328, 24.2418)
  line L714 (47.3328, 24.2418) -> (47.3917, 24.2722)
  line L715 (47.3917, 24.2722) -> (47.4533, 24.2999)
  line L716 (47.4533, 24.2999) -> (47.5176, 24.3248)
  line L717 (47.5176, 24.3248) -> (47.5848, 24.347)
  line L718 (47.5848, 24.347) -> (47.6547, 24.3663)
  line L719 (47.6547, 24.3663) -> (47.7275, 24.3828)
  line L720 (47.7275, 24.3828) -> (47.8033, 24.3964)
  line L721 (47.8033, 24.3964) -> (47.882, 24.407)
  line L722 (47.882, 24.407) -> (47.9636, 24.4146)
  line L723 (47.9636, 24.4146) -> (48.0483, 24.4192)
  line L724 (48.0483, 24.4192) -> (48.1361, 24.4207)
  line L725 (48.1361, 24.4207) -> (51.3111, 24.4207)
  line L726 (51.3111, 24.4207) -> (51.3988, 24.4192)
  line L727 (24.3587, 24.4192) -> (24.4442, 24.4146)
  line L728 (24.4442, 24.4146) -> (24.527, 24.407)
  line L729 (24.527, 24.407) -> (24.6072, 24.3964)
  line L730 (24.6072, 24.3964) -> (24.6845, 24.3828)
  line L731 (24.6845, 24.3828) -> (24.759, 24.3663)
  line L732 (24.759, 24.3663) -> (24.8305, 24.347)
  line L733 (24.8305, 24.347) -> (24.8991, 24.3248)
  line L734 (24.8991, 24.3248) -> (24.9645, 24.2999)
  line L735 (24.9645, 24.2999) -> (25.0267, 24.2722)
  line L736 (25.0267, 24.2722) -> (25.0857, 24.2418)
  line L737 (25.0857, 24.2418) -> (25.1413, 24.2087)
  line L738 (25.1413, 24.2087) -> (25.1935, 24.1729)
  line L739 (25.1935, 24.1729) -> (25.2423, 24.1346)
  line L740 (25.2423, 24.1346) -> (25.2875, 24.0937)
  line L741 (25.2875, 24.0937) -> (25.329, 24.0503)
  line L742 (25.329, 24.0503) -> (25.353, 24.0254)
  line L743 (25.353, 24.0254) -> (25.3756, 24.0002)
  line L744 (25.3756, 24.0002) -> (25.3967, 23.9748)
  line L745 (25.3967, 23.9748) -> (25.4163, 23.9493)
  line L746 (25.4163, 23.9493) -> (25.4347, 23.9237)
  line L747 (25.4347, 23.9237) -> (25.4517, 23.8982)
  line L748 (25.4517, 23.8982) -> (25.4674, 23.8727)
  line L749 (25.4674, 23.8727) -> (25.482, 23.8473)
  line L750 (25.482, 23.8473) -> (25.4953, 23.8222)
  line L751 (25.4953, 23.8222) -> (25.5076, 23.7973)
  line L752 (25.5076, 23.7973) -> (25.5188, 23.7727)
  line L753 (25.5188, 23.7727) -> (25.529, 23.7485)
  line L754 (25.529, 23.7485) -> (25.5465, 23.7015)
  line L755 (25.5465, 23.7015) -> (25.5605, 23.6568)
  line L756 (25.5605, 23.6568) -> (25.5714, 23.6148)
  line L757 (25.5714, 23.6148) -> (25.5796, 23.5762)
  line L758 (25.5796, 23.5762) -> (25.5855, 23.5414)
  line L759 (25.5855, 23.5414) -> (25.5895, 23.5108)
  line L760 (25.5895, 23.5108) -> (25.5918, 23.4851)
  line L761 (25.5918, 23.4851) -> (25.5931, 23.4647)
  line L762 (25.5931, 23.4647) -> (25.5936, 23.4418)
  line L763 (25.5936, 23.4418) -> (25.5936, 23.336)
  line L764 (25.5936, 23.336) -> (25.5931, 23.3131)
  line L765 (25.5931, 23.3131) -> (25.5895, 23.2673)
  line L766 (25.5895, 23.2673) -> (25.5855, 23.2372)
  line L767 (25.5855, 23.2372) -> (25.5796, 23.2029)
  line L768 (25.5796, 23.2029) -> (25.5714, 23.1651)
  line L769 (25.5714, 23.1651) -> (25.5605, 23.1243)
  line L770 (25.5605, 23.1243) -> (25.5465, 23.081)
  line L771 (25.5465, 23.081) -> (25.529, 23.0357)
  line L772 (25.529, 23.0357) -> (25.5076, 22.9891)
  line L773 (25.5076, 22.9891) -> (25.482, 22.9416)
  line L774 (25.482, 22.9416) -> (25.4517, 22.8937)
  line L775 (25.4517, 22.8937) -> (25.4347, 22.8699)
  line L776 (25.4347, 22.8699) -> (25.4163, 22.8462)
  line L777 (25.4163, 22.8462) -> (25.3967, 22.8226)
  line L778 (25.3967, 22.8226) -> (25.3756, 22.7994)
  line L779 (25.3756, 22.7994) -> (25.353, 22.7764)
  line L780 (25.353, 22.7764) -> (25.329, 22.7539)
  line L781 (25.329, 22.7539) -> (25.2889, 22.7142)
  line L782 (25.2889, 22.7142) -> (25.2681, 22.6943)
  line L783 (25.2681, 22.6943) -> (25.2463, 22.6745)
  line L784 (25.2463, 22.6745) -> (25.2233, 22.6546)
  line L785 (25.2233, 22.6546) -> (25.2113, 22.6447)
  line L786 (25.2113, 22.6447) -> (25.1988, 22.6348)
  line L787 (25.1988, 22.6348) -> (25.1858, 22.6249)
  line L788 (25.1858, 22.6249) -> (25.1724, 22.615)
  line L789 (25.1724, 22.615) -> (25.1584, 22.605)
  line L790 (25.1584, 22.605) -> (25.1438, 22.5951)
  line L791 (25.1438, 22.5951) -> (25.1584, 22.5852)
  line L792 (25.1584, 22.5852) -> (25.1724, 22.5753)
  line L793 (25.1724, 22.5753) -> (25.1858, 22.5654)
  line L794 (25.1858, 22.5654) -> (25.1988, 22.5554)
  line L795 (25.1988, 22.5554) -> (25.2113, 22.5455)
  line L796 (25.2113, 22.5455) -> (25.2233, 22.5356)
  line L797 (25.2233, 22.5356) -> (25.235, 22.5257)
  line L798 (25.235, 22.5257) -> (25.2463, 22.5157)
  line L799 (25.2463, 22.5157) -> (25.2681, 22.4959)
  line L800 (25.2681, 22.4959) -> (25.2889, 22.4761)
  line L801 (25.2889, 22.4761) -> (25.3091, 22.4562)
  line L802 (25.3091, 22.4562) -> (25.329, 22.4364)
  line L803 (25.329, 22.4364) -> (25.353, 22.4114)
  line L804 (25.353, 22.4114) -> (25.3756, 22.3862)
  line L805 (25.3756, 22.3862) -> (25.3967, 22.3608)
  line L806 (25.3967, 22.3608) -> (25.4163, 22.3353)
  line L807 (25.4163, 22.3353) -> (25.4347, 22.3098)
  line L808 (25.4347, 22.3098) -> (25.4517, 22.2842)
  line L809 (25.4517, 22.2842) -> (25.4674, 22.2587)
  line L810 (25.4674, 22.2587) -> (25.482, 22.2334)
  line L811 (25.482, 22.2334) -> (25.4953, 22.2082)
  line L812 (25.4953, 22.2082) -> (25.5076, 22.1833)
  line L813 (25.5076, 22.1833) -> (25.5188, 22.1587)
  line L814 (25.5188, 22.1587) -> (25.529, 22.1345)
  line L815 (25.529, 22.1345) -> (25.5465, 22.0875)
  line L816 (25.5465, 22.0875) -> (25.5605, 22.0428)
  line L817 (25.5605, 22.0428) -> (25.5714, 22.0009)
  line L818 (25.5714, 22.0009) -> (25.5796, 21.9622)
  line L819 (25.5796, 21.9622) -> (25.5855, 21.9274)
  line L820 (25.5855, 21.9274) -> (25.5895, 21.8969)
  line L821 (25.5895, 21.8969) -> (25.5918, 21.8711)
  line L822 (25.5918, 21.8711) -> (25.5931, 21.8507)
  line L823 (25.5931, 21.8507) -> (25.5936, 21.8278)
  line L824 (25.5936, 21.8278) -> (25.5936, 20.8753)
  line L825 (25.5936, 20.8753) -> (25.1438, 20.8753)
  line L826 (25.1438, 20.8753) -> (25.1438, 21.8278)
  line L827 (25.1438, 21.8278) -> (25.1421, 21.8506)
  line L828 (25.1421, 21.8506) -> (25.138, 21.8767)
  line L829 (25.138, 21.8767) -> (25.1302, 21.9105)
  line L830 (25.1302, 21.9105) -> (25.1171, 21.9506)
  line L831 (25.1171, 21.9506) -> (25.0978, 21.9953)
  line L832 (25.0978, 21.9953) -> (25.0707, 22.0431)
  line L833 (25.0707, 22.0431) -> (25.0539, 22.0676)
  line L834 (25.0539, 22.0676) -> (25.0347, 22.0924)
  line L835 (25.0347, 22.0924) -> (25.0129, 22.1172)
  line L836 (25.0129, 22.1172) -> (24.9884, 22.1418)
  line L837 (24.9884, 22.1418) -> (24.961, 22.166)
  line L838 (24.961, 22.166) -> (24.9306, 22.1896)
  line L839 (24.9306, 22.1896) -> (24.897, 22.2124)
  line L840 (24.897, 22.2124) -> (24.8601, 22.2343)
  line L841 (24.8601, 22.2343) -> (24.8196, 22.255)
  line L842 (24.8196, 22.255) -> (24.7754, 22.2743)
  line L843 (24.7754, 22.2743) -> (24.7275, 22.2921)
  line L844 (24.7275, 22.2921) -> (24.6755, 22.3082)
  line L845 (24.6755, 22.3082) -> (24.6193, 22.3223)
  line L846 (24.6193, 22.3223) -> (24.5589, 22.3343)
  line L847 (24.5589, 22.3343) -> (24.4939, 22.3439)
  line L848 (24.4939, 22.3439) -> (24.4244, 22.351)
  line L849 (24.4244, 22.351) -> (24.35, 22.3555)
  line L850 (24.35, 22.3555) -> (24.2707, 22.357)
  line L851 (24.2707, 22.357) -> (20.2225, 22.357)
  line L852 (20.2225, 22.357) -> (20.2225, 20.8753)
  line L853 (20.2225, 20.8753) -> (19.7728, 20.8753)
  line L854 (19.7728, 20.8753) -> (19.7728, 22.8068)
  line L855 (20.1961, 22.8068) -> (24.2442, 22.8068)
  line L856 (24.2442, 22.8068) -> (24.3075, 22.8074)
  line L857 (24.3075, 22.8074) -> (24.3683, 22.8094)
  line L858 (24.3683, 22.8094) -> (24.4267, 22.8127)
  line L859 (24.4267, 22.8127) -> (24.4827, 22.8175)
  line L860 (24.4827, 22.8175) -> (24.5365, 22.8239)
  line L861 (24.5365, 22.8239) -> (24.5879, 22.8319)
  line L862 (24.5879, 22.8319) -> (24.6371, 22.8416)
  line L863 (24.6371, 22.8416) -> (24.6841, 22.8531)
  line L864 (24.6841, 22.8531) -> (24.7289, 22.8664)
  line L865 (24.7289, 22.8664) -> (24.7716, 22.8817)
  line L866 (24.7716, 22.8817) -> (24.8122, 22.899)
  line L867 (24.8122, 22.899) -> (24.8507, 22.9184)
  line L868 (24.8507, 22.9184) -> (24.8872, 22.94)
  line L869 (24.8872, 22.94) -> (24.9217, 22.9638)
  line L870 (24.9217, 22.9638) -> (24.9543, 22.9899)
  line L871 (24.9543, 22.9899) -> (24.985, 23.0185)
  line L872 (24.985, 23.0185) -> (24.9995, 23.0286)
  line L873 (24.9995, 23.0286) -> (25.013, 23.0392)
  line L874 (25.013, 23.0392) -> (25.0256, 23.0501)
  line L875 (25.0256, 23.0501) -> (25.0374, 23.0613)
  line L876 (25.0374, 23.0613) -> (25.0484, 23.0729)
  line L877 (25.0484, 23.0729) -> (25.0586, 23.0846)
  line L878 (25.0586, 23.0846) -> (25.0681, 23.0965)
  line L879 (25.0681, 23.0965) -> (25.0768, 23.1086)
  line L880 (25.0768, 23.1086) -> (25.0848, 23.1207)
  line L881 (25.0848, 23.1207) -> (25.0922, 23.1328)
  line L882 (25.0922, 23.1328) -> (25.0989, 23.145)
  line L883 (25.0989, 23.145) -> (25.105, 23.157)
  line L884 (25.105, 23.157) -> (25.1106, 23.169)